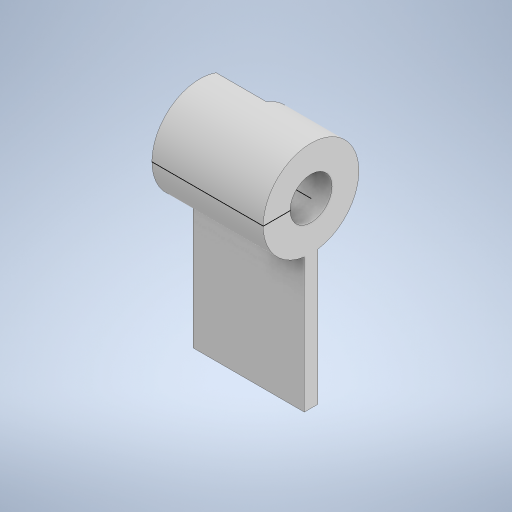
# Autodesk Inventor part: adjustable_collimator
Saved by Autodesk Inventor 2024 (Build 280153000, 153)
## iProperties
Created: 2025-02-06
Part Number: adjustable_collimator
Material: Generic
Document SubType Name: Modeling
Designer: Williamow
Density: 1 g/cm^3
Appearance: Default
Author: Williamow
Autodesk Inventor part; units mm, degrees
ref_plane "YZ Plane" through (0, 0, 0) normal (1, 0, 0) x (0, 1, 0)
ref_plane "XZ Plane" through (0, 0, 0) normal (0, 1, 0) x (-1, 0, 0)
ref_plane "XY Plane" through (0, 0, 0) normal (0, 0, 1) x (1, 0, 0)
sketch "Sketch1" plane through (0, 0, 0) normal (0, 1, 0) x (-1, 0, 0)
  line L0 (1.5, -2.15) -> (2.25, -2.15)
  line L1 (4.15, -2.96) -> (-1, -2.96)
  line L2 (-1, -2.96) -> (-1, -5)
  line L3 (0.8364, -2.3) -> (-2, -2.3)
  line L4 (-1, -5) -> (-2, -5)
  line L5 (-2, -5) -> (-2, -2.3)
  line L6 (-0.8, -0.5) -> (0.8364, -2.3)
  line L7 (0, 0) -> (-5, 0) construction
  line L8 (1.5, -2.15) -> (0, -0.5)
  line L9 (0, -0.5) -> (-0.8, -0.5)
  line L10 (2.25, -2.15) -> (3.25, -0.5)
  line L11 (3.25, -0.5) -> (4.05, -0.5)
  line L12 (4.05, -0.5) -> (4.15, -2.96)
  dimension "d0" = 2.3
  dimension "d4" = 2.15
  dimension "d5" = 0.75
  dimension "d9" = 0.81
  dimension "d10" = 1
  dimension "d11" = 5
  dimension "d22" = 0.8
  dimension "d27" = 0.8
  dimension "d45" = 3.5
  dimension "d47" = 1.5
  dimension "d48" = 0.1
  dimension "d54" = 0.5
  dimension "d55" = 1
  constraints: 26 end point, 5 horizontal, 2 horizontal alignment, 2 perpendicular, 1 parallel, 1 vertical alignment
  measures "d0" distance from line of L7.start L3
  measures "d4" distance from line of L7.start L0
  measures "d5" distance of L0.start L0.end
  measures "d9" distance between parallel lines of L1 L0
  measures "d10" distance of L2.end L4.end
  measures "d11" vertical distance of L4.end L7.start
  measures "d22" distance of L8.end L6.start
  measures "d27" distance of L10.end L11.end
  measures "d45" horizontal distance of L3.end L0.start
  measures "d47" horizontal distance of L7.start L0.start
  measures "d48" horizontal distance of L1.start L11.end
  measures "d54" vertical distance of L11.end L7.start
  measures "d55" horizontal distance of L0.end L10.end
sketch "Sketch4" plane through (0, 0, 0) normal (0, 1, 0) x (-1, 0, 0)
  line L0 (0, 1.25) -> (0, 2.85)
  line L1 (0, 2.85) -> (6.625, 2.85)
  line L2 (6.625, 2.85) -> (6.625, 1.25)
  line L3 (3.625, 0.5) -> (5.175, 2.05)
  line L4 (5.175, 2.05) -> (5.825, 2.05)
  line L5 (5.825, 2.05) -> (6.625, 1.25)
  line L6 (0, 1.25) -> (2, 1.25)
  line L7 (2, 1.25) -> (2.75, 0.5)
  line L8 (2.75, 0.5) -> (3.625, 0.5)
  line L9 (3.625, 0.5) -> (3.625, 2.85)
  line L10 (0, 0) -> (1.5, 0)
  point P0 (5.5, 2.05)
  dimension "d56" = 1.25
  dimension "d57" = 2
  dimension "d58" = 135
  dimension "d59" = 0.5
  dimension "d61" = 2.05
  dimension "d62" = 0.65
  dimension "d63" = 0.8
  dimension "d65" = 3.5
  dimension "d68" = 1.6
  constraints: 22 end point, 5 perpendicular, 3 horizontal, 1 midpoint, 1 parallel, 1 point on line, 1 vertical, 1 vertical alignment
  measures "d56" distance of L10.start L0.start
  measures "d57" distance of L0.start L6.end
  measures "d58" angle of L6 L7
  measures "d59" distance from line of L10.start L8
  measures "d61" distance from line of L10.start L4
  measures "d62" distance of L3.end L4.end
  measures "d63" distance between parallel lines of L1 L4
  measures "d65" horizontal distance of L6.end point (5.5, 2.05)
  measures "d68" distance of L1.end L2.end
revolve "Revolution5" add sketch "Sketch4" angle 360 about axis through (0, 0, 0) along (-1, 0, 0) contours L0 L1 L9 L8 L7 L6
revolve "Revolution6" add sketch "Sketch4" angle 220 mid plane about axis through (0, 0, 0) along (-1, 0, 0)
sketch "Sketch5" plane through (0, 0, 0) normal (1, 0, 0) x (0, 0, -1)
  circle A0 centre (0, 0) radius 2.85 projected
  line L0 (-0.4, 2.8218) -> (-0.4, 10.8218)
  line L1 (-0.4, 10.8218) -> (0.4, 10.8218)
  line L2 (0.4, 10.8218) -> (0.4, 2.8218)
  arc A1 (0.9748, 2.6781) -> (0.9748, -2.6781) centre (0, 0) ccw projected
  line L3 (-2.8218, -0.4) -> (-10.8218, -0.4)
  line L4 (-10.8218, -0.4) -> (-10.8218, 0.4)
  line L5 (-10.8218, 0.4) -> (-2.8218, 0.4)
  line L6 (-0.4, -2.8218) -> (-0.4, -10.8218)
  line L7 (-0.4, -10.8218) -> (0.4, -10.8218)
  line L8 (0.4, -10.8218) -> (0.4, -2.8218)
  point P0 (-2.8218, 0.4)
  point P1 (0.4, -2.8218)
  dimension "d69" = 0.8
  dimension "d70" = 8
  dimension "d15" = 1.2
  dimension "d30" = 1.2
  dimension "d31" = 1.2
  dimension "d34" = 3.5
  dimension "d50" = 120
  dimension "d51" = 0.8
  constraints: 18 end point, 6 equal length, 6 point on circle, 5 perpendicular, 3 vertical, 1 horizontal, 1 horizontal alignment
  measures "d69" distance of L0.end L1.end
  measures "d70" distance of L0.start L0.end
extrude "Extrusion5" add sketch "Sketch5" against normal up to surface (6.625 mm away) contours L8 L7 L6 A0
sketch "Sketch3" plane through (-9.15, 0, 0) normal (-1, 0, 0) x (0, 1, 0)
  arc A0 (1, 0.4583) -> (0, -1.1) centre (0, 0) ccw projected
  arc A1 (1, 0.4583) -> (0, -1.1) centre (0, 0) ccw projected
  arc A2 (1.0439, -0.3469) -> (-1.0439, -0.3469) centre (0, 2.5349) ccw
  arc A3 (0.6833, -0.8621) -> (-0.6833, -0.8621) centre (0, 2.5349) ccw
  circle A4 centre (0, 0) radius 6 projected
  dimension "d42" = 0.4
  constraints: 8 point on circle, 2 centre point, 1 coincident, 1 tangent, 1 vertical alignment
  measures "d42" radial gap between concentric circles of A3 A2
body "Solid1"
body "Solid3"
